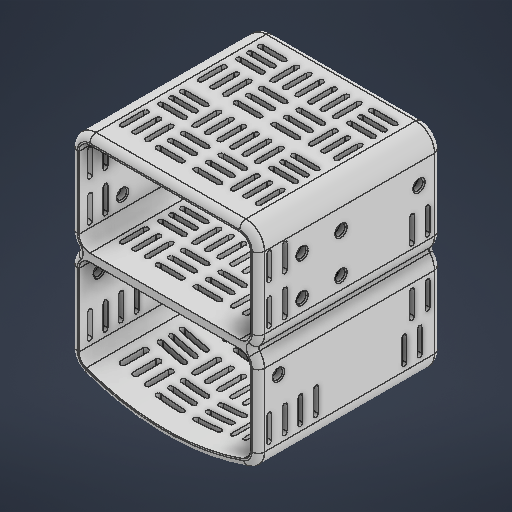
# Autodesk Inventor part: Корпус тела
Saved by Autodesk Inventor 2025 (Build 290162010, 162A)
## iProperties
Created: 2024-12-12
Part Number: Корпус тела
Material: Типовые
Document SubType Name: Modeling
Designer: Edward_Higgins
Density: 1 g/cm^3
Appearance: По умолчанию
Author: Edward_Higgins
Autodesk Inventor part; units mm, degrees
ref_plane "YZ Plane" through (0, 0, 0) normal (1, 0, 0) x (0, 1, 0)
ref_plane "XZ Plane" through (0, 0, 0) normal (0, 1, 0) x (-1, 0, 0)
ref_plane "XY Plane" through (0, 0, 0) normal (0, 0, 1) x (1, 0, 0)
sketch "Эскиз1" plane through (0, 0, 0) normal (0, 0, 1) x (1, 0, 0)
  line L0 (-55, 65) -> (-55, 19)
  line L1 (-48, 12) -> (48, 12)
  line L2 (48, 7) -> (-48, 7)
  line L3 (-55, 0) -> (-55, -46.4061)
  line L4 (55, -46.4061) -> (55, 0)
  arc A0 (48, 12) -> (55, 19) centre (48, 19) ccw
  arc A1 (-55, 19) -> (-48, 12) centre (-48, 19) ccw
  arc A2 (-48, 7) -> (-55, 0) centre (-48, 0) ccw
  arc A3 (55, 0) -> (48, 7) centre (48, 0) ccw
  line L5 (0, 167.0215) -> (0, -167.0215) construction
  line L6 (55, 19) -> (55, 65)
  arc A4 (-50.3497, -53) -> (50.3497, -53) centre (0, 88.2972) ccw
  arc A5 (-52.028, -57.7099) -> (52.028, -57.7099) centre (0, 88.2972) ccw
  line L7 (-48, 72) -> (48, 72)
  line L8 (48, 77) -> (-48, 77)
  arc A6 (-48, 72) -> (-55, 65) centre (-48, 65) ccw
  arc A7 (55, 65) -> (48, 72) centre (48, 65) ccw
  arc A8 (-48, 77) -> (-60, 65) centre (-48, 65) ccw
  arc A9 (60, 65) -> (48, 77) centre (48, 65) ccw
  arc A10 (-55, -46.4061) -> (-50.3497, -53) centre (-48, -46.4061) ccw
  arc A11 (50.3497, -53) -> (55, -46.4061) centre (48, -46.4061) ccw
  arc A12 (-60, -46.4061) -> (-52.028, -57.7099) centre (-48, -46.4061) ccw
  arc A13 (52.028, -57.7099) -> (60, -46.4061) centre (48, -46.4061) ccw
  arc A14 (-60, 19) -> (-55.3314, 9.5) centre (-48, 19) ccw
  arc A15 (-55.3314, 9.5) -> (-60, 0) centre (-48, 0) ccw
  arc A16 (55.3314, 9.5) -> (60, 19) centre (48, 19) ccw
  arc A17 (60, 0) -> (55.3314, 9.5) centre (48, 0) ccw
  line L9 (60, -46.4061) -> (60, 0)
  line L10 (60, 19) -> (60, 65)
  line L11 (-60, 65) -> (-60, 19)
  line L12 (-60, 0) -> (-60, -46.4061)
  point P0 (0, 0)
  point P1 (0, 7)
  point P2 (60, 0)
  point P3 (0, 0)
  dimension "d5" = 5
  dimension "d28" = 150
  dimension "d29" = 7
  dimension "d30" = 5
  dimension "d33" = 5
  dimension "d34" = 7
  dimension "d35" = 60
  dimension "d36" = 60
  dimension "d52" = 110
  constraints: 37 point on circle, 33 tangent, 27 end point, 18 centre point, 12 coincident, 9 equal radius, 7 parallel, 4 vertical alignment, 2 horizontal, 2 midpoint, 2 point on line, 1 horizontal alignment, 1 perpendicular, 1 vertical, 2 other
  measures "d5" distance between parallel lines of L2 L1
  measures "d28" radius of A4
  measures "d29" radius of A3
  measures "d30" distance between parallel lines of L10 L6
  measures "d33" radial gap between concentric circles of A4 A5
  measures "d34" distance from line of L2 point (0, 0)
  measures "d35" distance between parallel lines of L1 L7
  measures "d36" distance from line of L2 A4.start
  measures "d52" distance between parallel lines of L6 L0
extrude "Выдавливание1" add sketch "Эскиз1" along normal mid plane 117
sketch "Эскиз3" plane through (-60, -46.4061, 58.5) normal (-1, 0, 0) x (0, 0, 1)
  circle A0 centre (-28, 98.4061) radius 3.25
  circle A1 centre (-53, 98.4061) radius 3.25
  circle A2 centre (-28, 73.4061) radius 3.25
  circle A3 centre (-53, 73.4061) radius 3.25
  circle A4 centre (-13, 38.4061) radius 3.25
  circle A5 centre (-103, 98.4061) radius 3.25
  line L0 (0, 111.4061) -> (0, 65.4061) projected
  line L1 (-117, 123.4061) -> (0, 123.4061) projected
  point P0 (-58.5, 46.4061)
  dimension "d37" = 6.5
  dimension "d38" = 90
  dimension "d39" = 25
  dimension "d40" = 25
  dimension "d41" = 75
  dimension "d42" = 35
  dimension "d43" = 28
  dimension "d44" = 25
  constraints: 6 centre point, 5 equal radius, 3 horizontal alignment, 2 vertical alignment
  measures "d37" diameter of A5
  measures "d38" horizontal distance of A4.centre A5.centre
  measures "d39" distance of A2.centre A0.centre
  measures "d40" distance of A0.centre A1.centre
  measures "d41" distance of A5.centre A0.centre
  measures "d42" vertical distance of A4.centre A2.centre
  measures "d43" distance from line of L0 A0.centre
  measures "d44" distance from line of L1 A5.centre
extrude "Выдавливание2" cut sketch "Эскиз3" against normal up to surface (120 mm away)
fillet "Сопряжение1" radius 2 2 edges at (-55.3314, 9.5, 0) (55.3314, 9.5, 0)
fillet "Сопряжение2" radius 4 32 edges at (56.4853, 73.4853, 58.5) (0, 77, 58.5) (-56.4853, 73.4853, 58.5) (-60, 42, 58.5) (-59.1753, 14.6281, 58.5) (-56.2835, 9.5, 58.5) (-59.1753, 4.3719, 58.5) (-60, -23.2031, 58.5) (-57.8065, -53.3222, 58.5) (0, -66.7028, 58.5) (57.8065, -53.3222, 58.5) (60, -23.2031, 58.5) (59.1753, 4.3719, 58.5) (56.2835, 9.5, 58.5) (59.1753, 14.6281, 58.5) (60, 42, 58.5) (59.1753, 14.6281, -58.5) (56.2835, 9.5, -58.5) (59.1753, 4.3719, -58.5) (60, -23.2031, -58.5) (57.8065, -53.3222, -58.5) (0, -66.7028, -58.5) (-57.8065, -53.3222, -58.5) (-60, -23.2031, -58.5) (-59.1753, 4.3719, -58.5) (-56.2835, 9.5, -58.5) (-59.1753, 14.6281, -58.5) (-60, 42, -58.5) (-56.4853, 73.4853, -58.5) (0, 77, -58.5) (56.4853, 73.4853, -58.5) (60, 42, -58.5)
chamfer "Фаска1" distance 0.7 angle 45 24 edges at (-60, 52, -47.75) (-60, 52, 2.25) (-60, 52, 27.25) (-60, 27, 27.25) (-60, 27, 2.25) (-60, -8, 42.25) (55, -8, 42.25) (55, 27, 27.25) (55, 52, 27.25) (55, 52, 2.25) (55, 27, 2.25) (55, 52, -47.75) (60, 52, 27.25) (60, 52, 2.25) (60, 52, -47.75) (60, 27, 2.25) (60, 27, 27.25) (60, -8, 42.25) (-55, -8, 42.25) (-55, 27, 27.25) (-55, 27, 2.25) (-55, 52, 27.25) (-55, 52, 2.25) (-55, 52, -47.75)
sketch "Эскиз4" plane through (-48, 77, -54.5) normal (0, 1, 0) x (1, 0, 0)
  arc A0 (4.9257, -6.9474) -> (4.9257, -9.9474) centre (4.9257, -8.4474) ccw
  arc A1 (19.9257, -9.9474) -> (19.9257, -6.9474) centre (19.9257, -8.4474) ccw
  line L0 (4.9257, -6.9474) -> (19.9257, -6.9474)
  line L1 (19.9257, -9.9474) -> (4.9257, -9.9474)
  line L2 (48, 14.7293) -> (48, -124.0401) construction
  arc A2 (29.4257, -8.4474) -> (26.4257, -8.4474) centre (27.9257, -8.4474) ccw
  arc A3 (26.4257, -23.4474) -> (29.4257, -23.4474) centre (27.9257, -23.4474) ccw
  line L3 (29.4257, -8.4474) -> (29.4257, -23.4474)
  line L4 (26.4257, -8.4474) -> (26.4257, -23.4474)
  arc A4 (37.4257, -8.4474) -> (34.4257, -8.4474) centre (35.9257, -8.4474) ccw
  arc A5 (34.4257, -23.4474) -> (37.4257, -23.4474) centre (35.9257, -23.4474) ccw
  line L5 (37.4257, -8.4474) -> (37.4257, -23.4474)
  line L6 (34.4257, -8.4474) -> (34.4257, -23.4474)
  arc A6 (45.4257, -8.4474) -> (42.4257, -8.4474) centre (43.9257, -8.4474) ccw
  arc A7 (42.4257, -23.4474) -> (45.4257, -23.4474) centre (43.9257, -23.4474) ccw
  line L7 (45.4257, -8.4474) -> (45.4257, -23.4474)
  line L8 (42.4257, -8.4474) -> (42.4257, -23.4474)
  arc A8 (19.9257, -16.9474) -> (19.9257, -13.9474) centre (19.9257, -15.4474) ccw
  line L9 (4.9257, -13.9474) -> (19.9257, -13.9474)
  line L10 (19.9257, -16.9474) -> (4.9257, -16.9474)
  arc A9 (4.9257, -13.9474) -> (4.9257, -16.9474) centre (4.9257, -15.4474) ccw
  arc A10 (19.9257, -23.9474) -> (19.9257, -20.9474) centre (19.9257, -22.4474) ccw
  line L11 (4.9257, -20.9474) -> (19.9257, -20.9474)
  line L12 (19.9257, -23.9474) -> (4.9257, -23.9474)
  arc A11 (4.9257, -20.9474) -> (4.9257, -23.9474) centre (4.9257, -22.4474) ccw
  arc A12 (51.9257, -6.9474) -> (51.9257, -9.9474) centre (51.9257, -8.4474) ccw
  arc A13 (66.9257, -9.9474) -> (66.9257, -6.9474) centre (66.9257, -8.4474) ccw
  line L13 (51.9257, -6.9474) -> (66.9257, -6.9474)
  line L14 (66.9257, -9.9474) -> (51.9257, -9.9474)
  arc A14 (76.4257, -8.4474) -> (73.4257, -8.4474) centre (74.9257, -8.4474) ccw
  arc A15 (73.4257, -23.4474) -> (76.4257, -23.4474) centre (74.9257, -23.4474) ccw
  line L15 (76.4257, -8.4474) -> (76.4257, -23.4474)
  line L16 (73.4257, -8.4474) -> (73.4257, -23.4474)
  arc A16 (84.4257, -8.4474) -> (81.4257, -8.4474) centre (82.9257, -8.4474) ccw
  arc A17 (81.4257, -23.4474) -> (84.4257, -23.4474) centre (82.9257, -23.4474) ccw
  line L17 (84.4257, -8.4474) -> (84.4257, -23.4474)
  line L18 (81.4257, -8.4474) -> (81.4257, -23.4474)
  arc A18 (92.4257, -8.4474) -> (89.4257, -8.4474) centre (90.9257, -8.4474) ccw
  arc A19 (89.4257, -23.4474) -> (92.4257, -23.4474) centre (90.9257, -23.4474) ccw
  line L19 (92.4257, -8.4474) -> (92.4257, -23.4474)
  line L20 (89.4257, -8.4474) -> (89.4257, -23.4474)
  arc A20 (66.9257, -16.9474) -> (66.9257, -13.9474) centre (66.9257, -15.4474) ccw
  line L21 (51.9257, -13.9474) -> (66.9257, -13.9474)
  line L22 (66.9257, -16.9474) -> (51.9257, -16.9474)
  arc A21 (51.9257, -13.9474) -> (51.9257, -16.9474) centre (51.9257, -15.4474) ccw
  arc A22 (66.9257, -23.9474) -> (66.9257, -20.9474) centre (66.9257, -22.4474) ccw
  line L23 (51.9257, -20.9474) -> (66.9257, -20.9474)
  line L24 (66.9257, -23.9474) -> (51.9257, -23.9474)
  arc A23 (51.9257, -20.9474) -> (51.9257, -23.9474) centre (51.9257, -22.4474) ccw
  arc A24 (28.4257, -37.9489) -> (28.4257, -40.9489) centre (28.4257, -39.4489) ccw
  arc A25 (28.4257, -45.9489) -> (28.4257, -48.9489) centre (28.4257, -47.4489) ccw
  line L25 (28.4257, -29.9489) -> (43.4257, -29.9489)
  line L26 (43.4257, -32.9489) -> (28.4257, -32.9489)
  arc A26 (43.4257, -32.9489) -> (43.4257, -29.9489) centre (43.4257, -31.4489) ccw
  line L27 (28.4257, -37.9489) -> (43.4257, -37.9489)
  line L28 (43.4257, -40.9489) -> (28.4257, -40.9489)
  line L29 (28.4257, -45.9489) -> (43.4257, -45.9489)
  line L30 (43.4257, -48.9489) -> (28.4257, -48.9489)
  arc A27 (43.4257, -40.9489) -> (43.4257, -37.9489) centre (43.4257, -39.4489) ccw
  arc A28 (43.4257, -48.9489) -> (43.4257, -45.9489) centre (43.4257, -47.4489) ccw
  arc A29 (60.9257, -31.4489) -> (57.9257, -31.4489) centre (59.4257, -31.4489) ccw
  arc A30 (52.9257, -31.4489) -> (49.9257, -31.4489) centre (51.4257, -31.4489) ccw
  line L31 (57.9257, -31.4489) -> (57.9257, -46.4489)
  arc A31 (57.9257, -46.4489) -> (60.9257, -46.4489) centre (59.4257, -46.4489) ccw
  line L32 (52.9257, -31.4489) -> (52.9257, -46.4489)
  line L33 (49.9257, -31.4489) -> (49.9257, -46.4489)
  arc A32 (49.9257, -46.4489) -> (52.9257, -46.4489) centre (51.4257, -46.4489) ccw
  line L34 (60.9257, -31.4489) -> (60.9257, -46.4489)
  line L35 (65.9257, -31.4489) -> (65.9257, -46.4489)
  arc A33 (68.9257, -31.4489) -> (65.9257, -31.4489) centre (67.4257, -31.4489) ccw
  arc A34 (65.9257, -46.4489) -> (68.9257, -46.4489) centre (67.4257, -46.4489) ccw
  line L36 (68.9257, -31.4489) -> (68.9257, -46.4489)
  arc A35 (28.4257, -29.9489) -> (28.4257, -32.9489) centre (28.4257, -31.4489) ccw
  arc A36 (5.9257, -31.4489) -> (2.9257, -31.4489) centre (4.4257, -31.4489) ccw
  arc A37 (2.9257, -46.4489) -> (5.9257, -46.4489) centre (4.4257, -46.4489) ccw
  line L37 (5.9257, -31.4489) -> (5.9257, -46.4489)
  line L38 (2.9257, -31.4489) -> (2.9257, -46.4489)
  arc A38 (13.9257, -31.4489) -> (10.9257, -31.4489) centre (12.4257, -31.4489) ccw
  arc A39 (10.9257, -46.4489) -> (13.9257, -46.4489) centre (12.4257, -46.4489) ccw
  line L39 (13.9257, -31.4489) -> (13.9257, -46.4489)
  line L40 (10.9257, -31.4489) -> (10.9257, -46.4489)
  arc A40 (21.9257, -31.4489) -> (18.9257, -31.4489) centre (20.4257, -31.4489) ccw
  arc A41 (18.9257, -46.4489) -> (21.9257, -46.4489) centre (20.4257, -46.4489) ccw
  line L41 (21.9257, -31.4489) -> (21.9257, -46.4489)
  line L42 (18.9257, -31.4489) -> (18.9257, -46.4489)
  arc A42 (75.4257, -29.9489) -> (75.4257, -32.9489) centre (75.4257, -31.4489) ccw
  line L43 (75.4257, -29.9489) -> (90.4257, -29.9489)
  line L44 (90.4257, -32.9489) -> (75.4257, -32.9489)
  arc A43 (90.4257, -32.9489) -> (90.4257, -29.9489) centre (90.4257, -31.4489) ccw
  arc A44 (75.4257, -37.9489) -> (75.4257, -40.9489) centre (75.4257, -39.4489) ccw
  line L45 (90.4257, -40.9489) -> (75.4257, -40.9489)
  line L46 (75.4257, -37.9489) -> (90.4257, -37.9489)
  arc A45 (90.4257, -40.9489) -> (90.4257, -37.9489) centre (90.4257, -39.4489) ccw
  arc A46 (75.4257, -45.9489) -> (75.4257, -48.9489) centre (75.4257, -47.4489) ccw
  line L47 (90.4257, -48.9489) -> (75.4257, -48.9489)
  line L48 (75.4257, -45.9489) -> (90.4257, -45.9489)
  arc A47 (90.4257, -48.9489) -> (90.4257, -45.9489) centre (90.4257, -47.4489) ccw
  arc A48 (4.9257, -63.9474) -> (4.9257, -66.9474) centre (4.9257, -65.4474) ccw
  arc A49 (4.9257, -70.9474) -> (4.9257, -73.9474) centre (4.9257, -72.4474) ccw
  line L49 (4.9257, -56.9474) -> (19.9257, -56.9474)
  arc A50 (19.9257, -59.9474) -> (19.9257, -56.9474) centre (19.9257, -58.4474) ccw
  line L50 (19.9257, -59.9474) -> (4.9257, -59.9474)
  line L51 (4.9257, -63.9474) -> (19.9257, -63.9474)
  line L52 (19.9257, -66.9474) -> (4.9257, -66.9474)
  line L53 (4.9257, -70.9474) -> (19.9257, -70.9474)
  line L54 (19.9257, -73.9474) -> (4.9257, -73.9474)
  arc A51 (19.9257, -66.9474) -> (19.9257, -63.9474) centre (19.9257, -65.4474) ccw
  arc A52 (19.9257, -73.9474) -> (19.9257, -70.9474) centre (19.9257, -72.4474) ccw
  line L55 (48, -35.2707) -> (48, -174.0401) construction
  line L56 (42.4257, -58.4474) -> (42.4257, -73.4474)
  arc A53 (42.4257, -73.4474) -> (45.4257, -73.4474) centre (43.9257, -73.4474) ccw
  arc A54 (45.4257, -58.4474) -> (42.4257, -58.4474) centre (43.9257, -58.4474) ccw
  line L57 (45.4257, -58.4474) -> (45.4257, -73.4474)
  arc A55 (51.9257, -70.9474) -> (51.9257, -73.9474) centre (51.9257, -72.4474) ccw
  arc A56 (51.9257, -63.9474) -> (51.9257, -66.9474) centre (51.9257, -65.4474) ccw
  arc A57 (51.9257, -56.9474) -> (51.9257, -59.9474) centre (51.9257, -58.4474) ccw
  line L58 (66.9257, -59.9474) -> (51.9257, -59.9474)
  line L59 (66.9257, -66.9474) -> (51.9257, -66.9474)
  line L60 (51.9257, -63.9474) -> (66.9257, -63.9474)
  line L61 (66.9257, -73.9474) -> (51.9257, -73.9474)
  line L62 (51.9257, -70.9474) -> (66.9257, -70.9474)
  line L63 (51.9257, -56.9474) -> (66.9257, -56.9474)
  arc A58 (66.9257, -73.9474) -> (66.9257, -70.9474) centre (66.9257, -72.4474) ccw
  arc A59 (66.9257, -66.9474) -> (66.9257, -63.9474) centre (66.9257, -65.4474) ccw
  arc A60 (66.9257, -59.9474) -> (66.9257, -56.9474) centre (66.9257, -58.4474) ccw
  arc A61 (13.9257, -81.4489) -> (10.9257, -81.4489) centre (12.4257, -81.4489) ccw
  arc A62 (5.9257, -81.4489) -> (2.9257, -81.4489) centre (4.4257, -81.4489) ccw
  line L64 (2.9257, -81.4489) -> (2.9257, -96.4489)
  line L65 (5.9257, -81.4489) -> (5.9257, -96.4489)
  arc A63 (2.9257, -96.4489) -> (5.9257, -96.4489) centre (4.4257, -96.4489) ccw
  line L66 (10.9257, -81.4489) -> (10.9257, -96.4489)
  line L67 (13.9257, -81.4489) -> (13.9257, -96.4489)
  arc A64 (10.9257, -96.4489) -> (13.9257, -96.4489) centre (12.4257, -96.4489) ccw
  arc A65 (60.9257, -81.4489) -> (57.9257, -81.4489) centre (59.4257, -81.4489) ccw
  line L68 (57.9257, -81.4489) -> (57.9257, -96.4489)
  line L69 (60.9257, -81.4489) -> (60.9257, -96.4489)
  arc A66 (57.9257, -96.4489) -> (60.9257, -96.4489) centre (59.4257, -96.4489) ccw
  arc A67 (90.4257, -82.9489) -> (90.4257, -79.9489) centre (90.4257, -81.4489) ccw
  line L70 (75.4257, -79.9489) -> (90.4257, -79.9489)
  line L71 (90.4257, -82.9489) -> (75.4257, -82.9489)
  arc A68 (90.4257, -90.9489) -> (90.4257, -87.9489) centre (90.4257, -89.4489) ccw
  line L72 (75.4257, -87.9489) -> (90.4257, -87.9489)
  line L73 (90.4257, -90.9489) -> (75.4257, -90.9489)
  line L74 (75.4257, -95.9489) -> (90.4257, -95.9489)
  line L75 (90.4257, -98.9489) -> (75.4257, -98.9489)
  arc A69 (28.4257, -87.9489) -> (28.4257, -90.9489) centre (28.4257, -89.4489) ccw
  arc A70 (28.4257, -79.9489) -> (28.4257, -82.9489) centre (28.4257, -81.4489) ccw
  arc A71 (28.4257, -95.9489) -> (28.4257, -98.9489) centre (28.4257, -97.4489) ccw
  arc A72 (21.9257, -81.4489) -> (18.9257, -81.4489) centre (20.4257, -81.4489) ccw
  line L76 (21.9257, -81.4489) -> (21.9257, -96.4489)
  line L77 (18.9257, -81.4489) -> (18.9257, -96.4489)
  arc A73 (18.9257, -96.4489) -> (21.9257, -96.4489) centre (20.4257, -96.4489) ccw
  line L78 (43.4257, -98.9489) -> (28.4257, -98.9489)
  arc A74 (43.4257, -98.9489) -> (43.4257, -95.9489) centre (43.4257, -97.4489) ccw
  line L79 (28.4257, -95.9489) -> (43.4257, -95.9489)
  line L80 (49.9257, -81.4489) -> (49.9257, -96.4489)
  arc A75 (52.9257, -81.4489) -> (49.9257, -81.4489) centre (51.4257, -81.4489) ccw
  line L81 (52.9257, -81.4489) -> (52.9257, -96.4489)
  arc A76 (49.9257, -96.4489) -> (52.9257, -96.4489) centre (51.4257, -96.4489) ccw
  arc A77 (29.4257, -58.4474) -> (26.4257, -58.4474) centre (27.9257, -58.4474) ccw
  arc A78 (26.4257, -73.4474) -> (29.4257, -73.4474) centre (27.9257, -73.4474) ccw
  line L82 (29.4257, -58.4474) -> (29.4257, -73.4474)
  line L83 (37.4257, -58.4474) -> (37.4257, -73.4474)
  arc A79 (37.4257, -58.4474) -> (34.4257, -58.4474) centre (35.9257, -58.4474) ccw
  line L84 (34.4257, -58.4474) -> (34.4257, -73.4474)
  arc A80 (34.4257, -73.4474) -> (37.4257, -73.4474) centre (35.9257, -73.4474) ccw
  line L85 (26.4257, -58.4474) -> (26.4257, -73.4474)
  line L86 (65.9257, -81.4489) -> (65.9257, -96.4489)
  line L87 (68.9257, -81.4489) -> (68.9257, -96.4489)
  arc A81 (65.9257, -96.4489) -> (68.9257, -96.4489) centre (67.4257, -96.4489) ccw
  arc A82 (75.4257, -95.9489) -> (75.4257, -98.9489) centre (75.4257, -97.4489) ccw
  arc A83 (75.4257, -87.9489) -> (75.4257, -90.9489) centre (75.4257, -89.4489) ccw
  arc A84 (75.4257, -79.9489) -> (75.4257, -82.9489) centre (75.4257, -81.4489) ccw
  arc A85 (68.9257, -81.4489) -> (65.9257, -81.4489) centre (67.4257, -81.4489) ccw
  arc A86 (4.9257, -56.9474) -> (4.9257, -59.9474) centre (4.9257, -58.4474) ccw
  arc A87 (84.4257, -58.4474) -> (81.4257, -58.4474) centre (82.9257, -58.4474) ccw
  arc A88 (76.4257, -58.4474) -> (73.4257, -58.4474) centre (74.9257, -58.4474) ccw
  line L88 (81.4257, -58.4474) -> (81.4257, -73.4474)
  arc A89 (81.4257, -73.4474) -> (84.4257, -73.4474) centre (82.9257, -73.4474) ccw
  line L89 (76.4257, -58.4474) -> (76.4257, -73.4474)
  line L90 (73.4257, -58.4474) -> (73.4257, -73.4474)
  arc A90 (73.4257, -73.4474) -> (76.4257, -73.4474) centre (74.9257, -73.4474) ccw
  line L91 (84.4257, -58.4474) -> (84.4257, -73.4474)
  line L92 (89.4257, -58.4474) -> (89.4257, -73.4474)
  arc A91 (89.4257, -73.4474) -> (92.4257, -73.4474) centre (90.9257, -73.4474) ccw
  line L93 (92.4257, -58.4474) -> (92.4257, -73.4474)
  arc A92 (92.4257, -58.4474) -> (89.4257, -58.4474) centre (90.9257, -58.4474) ccw
  line L94 (43.4257, -90.9489) -> (28.4257, -90.9489)
  line L95 (28.4257, -87.9489) -> (43.4257, -87.9489)
  arc A93 (43.4257, -90.9489) -> (43.4257, -87.9489) centre (43.4257, -89.4489) ccw
  line L96 (43.4257, -82.9489) -> (28.4257, -82.9489)
  line L97 (28.4257, -79.9489) -> (43.4257, -79.9489)
  arc A94 (43.4257, -82.9489) -> (43.4257, -79.9489) centre (43.4257, -81.4489) ccw
  arc A95 (90.4257, -98.9489) -> (90.4257, -95.9489) centre (90.4257, -97.4489) ccw
  point P0 (48, -54.5)
  point P1 (35.9257, -29.9489)
  point P2 (59.4257, -23.9474)
  point P3 (12.4257, -23.9474)
  point P4 (82.9257, -29.9489)
  point P5 (82.9257, -37.9489)
  point P6 (82.9257, -45.9489)
  point P7 (12.4257, -73.9474)
  point P8 (48, -104.5)
  point P9 (59.4257, -73.9474)
  point P10 (82.9257, -79.9489)
  point P11 (82.9257, -87.9489)
  point P12 (82.9257, -95.9489)
  point P13 (35.9257, -79.9489)
  dimension "d53" = 3
  dimension "d54" = 15
  dimension "d57" = 8
  dimension "d62" = 8
  dimension "d65" = 7
  dimension "d78" = 3
  dimension "d79" = 15
  dimension "d80" = 8
  dimension "d81" = 8
  dimension "d82" = 7
  dimension "d93" = 3
  dimension "d94" = 15
  dimension "d95" = 8
  dimension "d96" = 8
  dimension "d97" = 8
  dimension "d100" = 8
  dimension "d101" = 5
  dimension "d102" = 3
  dimension "d103" = 15
  dimension "d106" = 8
  dimension "d113" = 50
  constraints: 196 end point, 192 point on circle, 96 centre point, 37 tangent, 12 vertical, 10 horizontal alignment, 8 vertical alignment, 7 equal radius, 7 horizontal, 5 parallel, 4 midpoint, 4 perpendicular, 2 point on line, 1 collinear, 391 other
  measures "d53" distance between parallel lines of L1 L0
  measures "d54" distance of A1.centre A0.centre
  measures "d57" distance of A2.centre A4.centre
  measures "d62" distance of A1.centre A2.centre
  measures "d65" distance of A1.centre A8.centre
  measures "d78" distance between parallel lines of L14 L13
  measures "d79" distance of A13.centre A12.centre
  measures "d80" distance of A14.centre A16.centre
  measures "d81" distance of A13.centre A14.centre
  measures "d82" distance of A13.centre A20.centre
  measures "d93" distance between parallel lines of L26 L25
  measures "d94" distance of A26.centre A35.centre
  measures "d95" distance of A30.centre A29.centre
  measures "d96" distance of A26.centre A30.centre
  measures "d97" distance of A26.centre A27.centre
  measures "d100" distance of A36.centre A38.centre
  measures "d101" distance between parallel lines of L39 L42
  measures "d102" distance between parallel lines of L44 L43
  measures "d103" distance of A43.centre A42.centre
  measures "d106" distance of L43.start L46.start
  measures "d113" distance of L9.start L51.start
extrude "Выдавливание3" cut sketch "Эскиз4" against normal up to surface contours L0 A1 L1 A0 | L3 A3 L4 A2 | L5 A5 L6 A4 | L7 A7 L8 A6 | L10 A9 L9 A8 | L12 A11 L11 A10 | L27 A27 L28 A24 | L29 A28 L30 A25 | L25 A26 L26 A35 | L37 A37 L38 A36 | L39 A39 L40 A38 | L41 A41 L42 A40 | L51 A51 L52 A48 | L53 A52 L54 A49 | L49 A50 L50 A86 | A54 L57 A53 L56 | L67 A64 L66 A61 | L65 A63 L64 A62 | L95 A93 L94 A69 | L97 A94 L96 A70 | L79 A74 L78 A71 | L76 A73 L77 A72 | L82 A78 L85 A77 | L83 A80 L84 A79 round surface about axis through (0, 88.2972, 0) along (0, 0, 1) radius 155 far side no
sketch "Эскиз5" plane through (60, -46.4061, -54.5) normal (1, 0, 0) x (0, 0, -1)
  arc A0 (-3, 42.3225) -> (-6, 42.3225) centre (-4.5, 42.3225) ccw
  arc A1 (-6, 27.3225) -> (-3, 27.3225) centre (-4.5, 27.3225) ccw
  line L0 (-3, 42.3225) -> (-3, 27.3225)
  line L1 (-6, 42.3225) -> (-6, 27.3225)
  arc A2 (-3, 83.606) -> (-6, 83.606) centre (-4.5, 83.606) ccw
  arc A3 (-6, 68.606) -> (-3, 68.606) centre (-4.5, 68.606) ccw
  line L2 (-3, 83.606) -> (-3, 68.606)
  line L3 (-6, 83.606) -> (-6, 68.606)
  arc A4 (-104.5, 108.9971) -> (-107.5, 108.9971) centre (-106, 108.9971) ccw
  arc A5 (-107.5, 93.9971) -> (-104.5, 93.9971) centre (-106, 93.9971) ccw
  line L4 (-104.5, 108.9971) -> (-104.5, 93.9971)
  line L5 (-107.5, 108.9971) -> (-107.5, 93.9971)
  arc A6 (-104.5, 83.606) -> (-107.5, 83.606) centre (-106, 83.606) ccw
  arc A7 (-107.5, 68.606) -> (-104.5, 68.606) centre (-106, 68.606) ccw
  line L6 (-104.5, 83.606) -> (-104.5, 68.606)
  line L7 (-107.5, 83.606) -> (-107.5, 68.606)
  arc A8 (-104.5, 19.1244) -> (-107.5, 19.1244) centre (-106, 19.1244) ccw
  arc A9 (-107.5, 4.1244) -> (-104.5, 4.1244) centre (-106, 4.1244) ccw
  line L8 (-104.5, 19.1244) -> (-104.5, 4.1244)
  line L9 (-107.5, 19.1244) -> (-107.5, 4.1244)
  arc A10 (-8, 19.1244) -> (-11, 19.1244) centre (-9.5, 19.1244) ccw
  arc A11 (-11, 4.1244) -> (-8, 4.1244) centre (-9.5, 4.1244) ccw
  line L10 (-8, 19.1244) -> (-8, 4.1244)
  line L11 (-11, 19.1244) -> (-11, 4.1244)
  line L12 (-54.5, 46.4061) -> (25.6207, 46.4061)
  line L13 (-21, 19.1244) -> (-21, 4.1244)
  arc A12 (-21, 4.1244) -> (-18, 4.1244) centre (-19.5, 4.1244) ccw
  line L14 (-18, 19.1244) -> (-18, 4.1244)
  arc A13 (-18, 19.1244) -> (-21, 19.1244) centre (-19.5, 19.1244) ccw
  arc A14 (-16, 27.3225) -> (-13, 27.3225) centre (-14.5, 27.3225) ccw
  line L15 (-16, 42.3225) -> (-16, 27.3225)
  line L16 (-13, 42.3225) -> (-13, 27.3225)
  arc A15 (-13, 42.3225) -> (-16, 42.3225) centre (-14.5, 42.3225) ccw
  arc A16 (-16, 68.606) -> (-13, 68.606) centre (-14.5, 68.606) ccw
  line L17 (-16, 83.606) -> (-16, 68.606)
  line L18 (-13, 83.606) -> (-13, 68.606)
  arc A17 (-13, 83.606) -> (-16, 83.606) centre (-14.5, 83.606) ccw
  line L19 (4, 0) -> (4, 46.4061) projected
  line L20 (-113, 111.4061) -> (-113, 65.4061) projected
  dimension "d120" = 15
  dimension "d122" = 3
  dimension "d123" = 15
  dimension "d124" = 3
  dimension "d125" = 15
  dimension "d126" = 3
  dimension "d127" = 15
  dimension "d128" = 3
  dimension "d129" = 15
  dimension "d130" = 3
  dimension "d131" = 15
  dimension "d132" = 3
  dimension "d135" = 10
  dimension "d140" = 7
  dimension "d141" = 5
  dimension "d142" = 7
  constraints: 38 end point, 36 point on circle, 18 centre point, 12 parallel, 12 tangent, 6 equal radius, 6 vertical, 3 vertical alignment, 2 horizontal, 30 other
  measures "d120" distance of A1.centre A0.centre
  measures "d122" distance between parallel lines of L0 L1
  measures "d123" distance of A3.centre A2.centre
  measures "d124" distance between parallel lines of L2 L3
  measures "d125" distance of A5.centre A4.centre
  measures "d126" distance between parallel lines of L4 L5
  measures "d127" distance of A7.centre A6.centre
  measures "d128" distance between parallel lines of L6 L7
  measures "d129" distance of A9.centre A8.centre
  measures "d130" distance between parallel lines of L8 L9
  measures "d131" distance of A11.centre A10.centre
  measures "d132" distance between parallel lines of L10 L11
  measures "d135" distance of L11.end L13.end
  measures "d140" distance between parallel lines of L19 L0
  measures "d141" horizontal distance of A1.centre A10.centre
  measures "d142" distance from line of L20 A7.centre
extrude "Выдавливание4" cut sketch "Эскиз5" against normal up to surface (120 mm away) contours L0 A1 L1 A0 | L2 A3 L3 A2 | L10 A11 L11 A10 | A13 L14 A12 L13 | L15 A15 L16 A14 | L17 A17 L18 A16
extrude "Выдавливание5" cut sketch "Эскиз5" against normal up to surface (120 mm away) contours L4 A5 L5 A4 | L6 A7 L7 A6
pattern_linear "Прямоуг.массив1" count 2 spacing 10 along (0, 0, -1) of "Выдавливание5"
extrude "Выдавливание6" cut sketch "Эскиз5" against normal up to surface (120 mm away) contours L8 A9 L9 A8
pattern_linear "Прямоуг.массив2" count 4 spacing 10 along (0, 0, -1) of "Выдавливание6"
mirror "Зеркальное отражение1" about plane through (0, 0, 0) normal (1, 0, 0) of "Выдавливание3"
equation "\"d5\" = d3"
equation "\"d3\" = 5"
